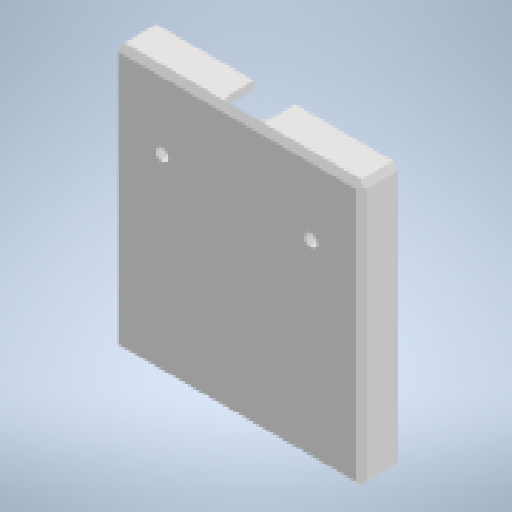
# Autodesk Inventor part: Bottom
Saved by Autodesk Inventor 2023.1 (Build 271208000, 208)
## iProperties
Created: 2023-03-16
Part Number: Bottom
Material: Generisch
Document SubType Name: Modeling
Designer: nikla
Density: 1 g/cm^3
Appearance: Vorgabe
Author: nikla
Autodesk Inventor part; units mm, degrees
ref_plane "YZ Plane" through (0, 0, 0) normal (1, 0, 0) x (0, 1, 0)
ref_plane "XZ Plane" through (0, 0, 0) normal (0, 1, 0) x (-1, 0, 0)
ref_plane "XY Plane" through (0, 0, 0) normal (0, 0, 1) x (1, 0, 0)
sketch "Skizze1" plane through (0, 0, 0) normal (0, 0, 1) x (1, 0, 0)
  line L0 (-39.95, 42.95) -> (-39.95, -42.95) projected
  line L1 (-39.95, -42.95) -> (39.95, -42.95) projected
  line L2 (39.95, -42.95) -> (39.95, 42.95) projected
  line L3 (39.95, 42.95) -> (-39.95, 42.95) projected
  line L4 (-36.95, 39.95) -> (-15, 39.95)
  line L5 (36.95, 39.95) -> (36.95, -39.95)
  line L6 (36.95, -39.95) -> (-36.95, -39.95)
  line L7 (-36.95, -39.95) -> (-36.95, 39.95)
  line L8 (-36.95, 39.95) -> (36.95, -39.95) construction
  line L9 (36.95, 39.95) -> (-36.95, -39.95) construction
  line L10 (0, -67.13) -> (0, 67.13) projected
  line L11 (-15, 39.95) -> (-15, 42.95)
  line L12 (15, 39.95) -> (15, 42.95)
  line L13 (15, 39.95) -> (36.95, 39.95)
  line L14 (44.95, -47.95) -> (-44.95, -47.95)
  line L15 (-44.95, -47.95) -> (-44.95, 47.95)
  line L16 (-44.95, 47.95) -> (-15, 47.95)
  line L17 (44.95, 47.95) -> (44.95, -47.95)
  line L18 (44.95, -47.95) -> (-44.95, 47.95) construction
  line L19 (-44.95, -47.95) -> (44.95, 47.95) construction
  line L20 (-15, 42.95) -> (-15, 47.95)
  line L21 (15, 42.95) -> (15, 47.95)
  line L22 (15, 47.95) -> (44.95, 47.95)
  point P0 (0, 0)
  point P1 (-15, 41.45)
  dimension "d0" = 3
  dimension "d1" = 3
  dimension "d2" = 30
  dimension "d4" = 5
  dimension "d5" = 5
  constraints: 36 end point, 6 parallel, 6 perpendicular, 5 midpoint, 3 horizontal, 3 symmetric about line, 1 point on line
  measures "d0" distance between parallel lines of L1 L6
  measures "d1" distance between parallel lines of L0 L7
  measures "d2" diameter of point (-15, 41.45) L10
  measures "d4" distance between parallel lines of L15 L0
  measures "d5" distance between parallel lines of L14 L1
extrude "Extrusion1" add sketch "Skizze1" along normal blind 10 contours L3 L11 L4 L7 L6 L10 L1 L0 | L0 L1 L10 L14 L15 L16 L20 L3 | L10 L6 L5 L13 L12 L3 L2 L1 | L1 L2 L3 L21 L22 L17 L14 L10
sketch "Skizze2" plane through (0, 0, 0) normal (0, 0, -1) x (-1, 0, 0)
  line L0 (-39.95, 42.95) -> (39.95, 42.95) projected
  line L1 (39.95, 42.95) -> (39.95, -42.95) projected
  line L2 (39.95, -42.95) -> (-39.95, -42.95) projected
  line L3 (-39.95, -42.95) -> (-39.95, 42.95) projected
  line L4 (-44.95, -47.95) -> (-44.95, 47.95) projected
  line L5 (-44.95, 47.95) -> (-15, 47.95) projected
  line L6 (44.95, -47.95) -> (-44.95, -47.95) projected
  line L7 (44.95, 47.95) -> (44.95, -47.95) projected
  line L8 (15, 47.95) -> (44.95, 47.95) projected
  line L9 (15, 39.95) -> (15, 47.95) projected
  line L10 (15, 47.95) -> (44.95, 47.95) projected
  line L11 (15, 47.95) -> (15, 42.95)
  line L12 (15, 39.95) -> (15, 47.95) projected
  line L13 (15, 47.95) -> (44.95, 47.95)
  line L14 (44.95, 47.95) -> (44.95, -47.95) projected
  line L15 (44.95, -47.95) -> (44.95, 47.95)
  line L16 (15, 42.95) -> (39.95, 42.95)
  line L17 (39.95, 42.95) -> (39.95, -42.95)
  line L18 (39.95, -42.95) -> (-39.95, -42.95)
  line L19 (-39.95, 42.95) -> (-39.95, -42.95)
  line L20 (-39.95, 42.95) -> (-15, 42.95)
  line L21 (-15, 47.95) -> (-15, 39.95) projected
  line L22 (-15, 42.95) -> (-15, 47.95)
  line L23 (-44.95, -47.95) -> (-44.95, 47.95) projected
  line L24 (-15, 47.95) -> (-44.95, 47.95)
  line L25 (-44.95, 47.95) -> (-44.95, -47.95)
  point P0 (0, 0)
  constraints: 22 end point, 4 collinear, 4 perpendicular, 4 point on line, 1 horizontal
extrude "Extrusion2" add sketch "Skizze2" along normal blind 1.6 contours L3 L2 L1 L0 L9 L8 L7 L6 L4 L5 L21
sketch "Skizze3" plane through (0, 0, 10) normal (0, 0, 1) x (1, 0, 0)
  line L0 (44.95, -47.95) -> (-44.95, -47.95) projected
  line L1 (-44.95, 47.95) -> (44.95, 47.95)
  line L2 (44.95, 47.95) -> (44.95, -47.95)
  line L3 (44.95, -47.95) -> (-44.95, -47.95)
  line L4 (-44.95, -47.95) -> (-44.95, 47.95)
  point P0 (0, 0)
  constraints: 8 end point, 2 parallel, 1 horizontal, 1 perpendicular
extrude "Extrusion3" add sketch "Skizze3" along normal blind 2
sketch "Skizze4" plane through (0, 0, 10) normal (0, 0, -1) x (-1, 0, 0)
  line L0 (15, 39.95) -> (15, 47.95) projected
  line L1 (-15, 47.95) -> (15, 47.95) projected
  line L2 (-15, 47.95) -> (-15, 39.95) projected
  line L3 (-15, 39.95) -> (-36.95, 39.95) projected
  line L4 (-36.95, 39.95) -> (-36.95, -39.95) projected
  line L5 (-36.95, -39.95) -> (36.95, -39.95) projected
  line L6 (36.95, -39.95) -> (36.95, 39.95) projected
  line L7 (36.95, 39.95) -> (15, 39.95) projected
  line L8 (0, -67.13) -> (0, 67.13) projected
  line L9 (-15, 47.95) -> (15, 47.95) projected
  line L10 (15, 47.95) -> (7.5, 47.95)
  line L11 (7.5, 47.95) -> (7.5, 44.95)
  line L12 (7.5, 44.95) -> (15, 44.95)
  line L13 (15, 44.95) -> (15, 47.95)
  line L14 (-15, 39.95) -> (-15, 47.95)
  line L15 (15, 47.95) -> (-15, 47.95)
  line L16 (-7.5, 47.95) -> (-7.5, 44.95)
  line L17 (-7.5, 44.95) -> (-15, 44.95)
  point P0 (0, 0)
  point P1 (-7.5, 47.95)
  point P2 (-15, 44.95)
  point P3 (15, 44.95)
  point P4 (7.5, 47.95)
  point P5 (7.5, 46.45)
  point P6 (11.25, 47.95)
  dimension "d14" = 15
  dimension "d15" = 3
  constraints: 16 end point, 5 symmetric about line, 2 midpoint, 2 parallel, 1 horizontal, 1 perpendicular
  measures "d14" distance from line of L16 point (7.5, 46.45)
  measures "d15" distance from line of point (11.25, 47.95) L12
extrude "Extrusion4" add sketch "Skizze4" along normal up to surface (11.6 mm away) contours L12 L11 L1 L0 | L16 L17 L2 L1
fillet "Rundung1" radius 2 2 edges at (-7.5, 46.45, 10) (7.5, 46.45, 10)
fillet "Rundung2" [suppressed]
fillet "Rundung3" [suppressed]
sketch "Skizze5" plane through (0, 0, 10) normal (0, 0, -1) x (-1, 0, 0)
  circle A0 centre (-26.75, 21.7) radius 1.1 projected
  circle A1 centre (27.25, 21.65) radius 1.1 projected
  point P0 (0, 0)
extrude "Extrusion5" cut sketch "Skizze5" against normal through all
sketch "Skizze6" plane through (0, 0, 10) normal (0, 0, -1) x (-1, 0, 0)
  point P0 (0, 0)
sketch "Skizze7" plane through (0, 0, 10) normal (0, 0, -1) x (-1, 0, 0)
  circle A0 centre (27.25, 21.65) radius 1.1 projected
  circle A1 centre (-26.75, 21.7) radius 1.1 projected
  line L0 (-5.5, 44.95) -> (-5.5, 47.95) projected
  line L1 (-5.5, 44.95) -> (-15, 44.95) projected
  line L2 (-15, 44.95) -> (-15, 39.95) projected
  line L3 (-15, 39.95) -> (-36.95, 39.95) projected
  line L4 (-36.95, 39.95) -> (-36.95, -39.95) projected
  line L5 (-36.95, -39.95) -> (36.95, -39.95) projected
  line L6 (36.95, -39.95) -> (36.95, 39.95) projected
  line L7 (36.95, 39.95) -> (15, 39.95) projected
  line L8 (15, 39.95) -> (15, 44.95) projected
  line L9 (15, 44.95) -> (5.5, 44.95) projected
  line L10 (5.5, 47.95) -> (5.5, 44.95) projected
  circle A2 centre (27.25, 21.65) radius 1.1 projected
  circle A3 centre (27.25, 21.65) radius 4.5
  line L11 (0, -67.1304) -> (0, 67.1322) projected
  circle A4 centre (-26.75, 21.7) radius 4.5
  line L12 (-5.5, 47.95) -> (5.5, 47.95) projected
  point P0 (0, 0)
  dimension "d21" = 9
  constraints: 2 centre point, 2 coincident
  measures "d21" diameter of A3
extrude "Extrusion6" add sketch "Skizze7" along normal blind 6 contours A3 | A4
sketch "Skizze8" plane through (0, 0, 12) normal (0, 0, 1) x (1, 0, 0)
  line L0 (0, -67.1304) -> (0, 67.1322) projected
  circle A0 centre (-27.25, 21.65) radius 1.1 projected
  circle A1 centre (-27.25, 21.65) radius 2.25
  circle A2 centre (26.75, 21.7) radius 1.1 projected
  circle A3 centre (26.75, 21.7) radius 2.25
  point P0 (0, 0)
  dimension "d24" = 4.5
  dimension "d25" = 4.5
  constraints: 2 centre point, 2 coincident
  measures "d24" diameter of A1
  measures "d25" diameter of A3
extrude "Extrusion7" cut sketch "Skizze8" against normal blind 3
chamfer "Fase1" distance 2 angle 45 4 edges at (44.95, 0, 12) (0, -47.95, 12) (0, 47.95, 12) (-44.95, 0, 12)
chamfer "Fase2" distance 2 angle 45 4 edges at (-44.95, 47.95, 4.2) (-44.95, -47.95, 4.2001) (44.95, -47.95, 4.2001) (44.95, 47.95, 4.2)
